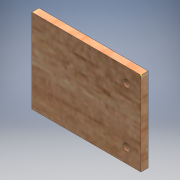
# Autodesk Inventor part: FrontSupport
Saved by Autodesk Inventor 2016 (Build 200138000, 138)
## iProperties
Created: 2016-04-01
Part Number: FrontSupport
Material: Wood (Birch)
Document SubType Name: Modeling
Designer: mkepler
Mass: 2.62763 g
Surface Area: 36.68 cm^2
Volume: 4.7775 cm^3
Density: 0.55 g/cm^3
Appearance: Birch - Natural Polished
Author: mkepler
Autodesk Inventor part; units mm, degrees
ref_plane "YZ Plane" through (0, 0, 0) normal (1, 0, 0) x (0, 1, 0)
ref_plane "XZ Plane" through (0, 0, 0) normal (0, 1, 0) x (-1, 0, 0)
ref_plane "XY Plane" through (0, 0, 0) normal (0, 0, 1) x (1, 0, 0)
sketch "Sketch1" plane through (0, 0, 0) normal (0, 1, 0) x (-1, 0, 0)
  point P0 (0, 0)
sketch "Sketch2" plane through (0, 0, 0) normal (0, 1, 0) x (-1, 0, 0)
  line L0 (0, 0) -> (45.5, 0)
  line L1 (45.5, 0) -> (45.5, -35)
  line L2 (45.5, -35) -> (0, -35)
  line L3 (0, -35) -> (0, 0)
  dimension "d0" = 45.5
  dimension "d1" = 35
  constraints: 8 end point, 2 parallel, 1 horizontal, 1 perpendicular
  measures "d0" distance of L1.end L2.end
  measures "d1" distance of L0.end L1.end
extrude "Extrusion1" add sketch "Sketch2" along normal blind 3
sketch "Sketch3" plane through (0, 3, 0) normal (0, 1, 0) x (1, 0, 0)
  circle A0 centre (-6, 6) radius 1
  line L0 (-45.5, 0) -> (0, 0) projected
  line L1 (0, 0) -> (0, 35) projected
  circle A1 centre (-6, 29) radius 1
  line L2 (0, 35) -> (-45.5, 35) projected
  dimension "d4" = 2
  dimension "d5" = 6
  dimension "d6" = 6
  dimension "d7" = 2
  dimension "d8" = 6
  dimension "d9" = 6
  constraints: 2 centre point
  measures "d4" diameter of A0
  measures "d5" distance from line of L0 A0.centre
  measures "d6" distance from line of L1 A0.centre
  measures "d7" diameter of A1
  measures "d8" distance from line of L2 A1.centre
  measures "d9" distance from line of L1 A1.centre
hole "Hole1" at (-6, 3, -6) at (-6, 3, -29) direction (0, -1, 0) diameter 3 end through all
body "Solid1"
